Autodesk Fusion 360 part; units mm, degrees
(part 2 of 2)
sketch "Sketch14" plane through (0, 0, 0) normal (0, 0, 1) x (-1, 0, 0)
  spline S0 degree 5 poles (1.1125, -9.059) (1.0978, -9.0455) (1.0555, -9.011) (1.011, -8.9912) (0.9641, -8.9931) (0.9095, -9.0155) (0.8665, -9.0398) (0.8607, -9.0432) knots 0.525573 0.525573 0.525573 0.525573 0.525573 0.525573 0.528205 0.533333 0.534119 0.534119 0.534119 0.534119 0.534119 0.534119
  arc A0 (1.1125, -9.059) -> (0.8607, -9.0432) centre (0.8856, -10.654) ccw
  arc A1 (-0.4184, -9.7079) -> (2.3934, -10.0866) centre (0.8856, -10.654) ccw
  spline S1 degree 5 poles (0.6709, 13.445) (0.783, 13.4498) (1.0072, 13.459) (1.3442, 13.4715) (1.7958, 13.4859) (2.365, 13.4975) (2.9391, 13.4984) (3.5187, 13.4833) (4.106, 13.4469) (4.7062, 13.3844) (5.3283, 13.2926) (5.9822, 13.1694) (6.6768, 13.0129) (7.4173, 12.8216) (8.2027, 12.5932) (9.0235, 12.3247) (9.8597, 12.0116) (10.6769, 11.6473) (11.4304, 11.2245) (12.0725, 10.7371) (12.5591, 10.1826) (12.8561, 9.5641) (12.9463, 8.892) (12.8356, 8.1865) (12.5616, 7.4801) (12.1923, 6.8157) (11.8085, 6.235) (11.4898, 5.7696) (11.2987, 5.4297) (11.2671, 5.1966) (11.3773, 5.0079) (11.5611, 4.7626) (11.7362, 4.3632) (11.8325, 3.7477) (11.8251, 2.9297) (11.7255, 1.9782) (11.5691, 0.9945) (11.4045, 0.0892) (11.2826, -0.6397) (11.2442, -1.1314) (11.3109, -1.3806) (11.4696, -1.4712) (11.6758, -1.5583) (11.8871, -1.7597) (12.0894, -2.0706) (12.2879, -2.4194) (12.4965, -2.7197) (12.728, -2.9335) (12.9875, -3.0981) (13.2749, -3.2834) (13.5856, -3.566) (13.912, -3.9925) (14.2441, -4.5797) (14.5698, -5.3213) (14.8753, -6.1921) (15.1462, -7.1536) (15.3673, -8.1587) (15.5233, -9.1573) (15.5998, -10.1003) (15.5828, -10.9464) (15.4608, -11.6626) (15.2255, -12.2237) (14.8731, -12.6119) (14.4066, -12.8168) (13.8357, -12.8345) (13.1799, -12.6674) (12.4665, -12.3245) (11.7278, -11.8208) (10.9984, -11.1782) (10.3118, -10.4256) (9.698, -9.5988) (9.1805, -8.7406) (8.7731, -7.9018) (8.4778, -7.1402) (8.2807, -6.5221) (8.1557, -6.1073) (8.0671, -5.9319) (7.9735, -5.9948) (7.8294, -6.2361) (7.593, -6.5406) (7.2472, -6.7929) (6.8148, -6.9181) (6.383, -6.9377) (6.0614, -6.9338) (5.9338, -7.0029) (6.0018, -7.2066) (6.1645, -7.543) (6.2897, -7.972) (6.2688, -8.4304) (6.0758, -8.8508) (5.7419, -9.1752) (5.3303, -9.3696) (4.9133, -9.4359) (4.5448, -9.4322) (4.2529, -9.4431) (4.0374, -9.5402) (3.8635, -9.7382) (3.6665, -9.976) (3.3863, -10.167) (3.0517, -10.228) (2.7549, -10.1966) (2.5418, -10.1395) (2.4216, -10.0971) (2.3934, -10.0866) knots 0 0 0 0 0 0 0.00512821 0.01025641 0.01538462 0.02051282 0.02564103 0.03076923 0.03589744 0.04102564 0.04615385 0.05128205 0.05641026 0.06153846 0.06666667 0.07179487 0.07692308 0.08205128 0.08717949 0.09230769 0.0974359 0.1025641 0.10769231 0.11282051 0.11794872 0.12307692 0.12820513 0.13333333 0.13846154 0.14358974 0.14871795 0.15384615 0.15897436 0.16410256 0.16923077 0.17435897 0.17948718 0.18461538 0.18974359 0.19487179 0.2 0.20512821 0.21025641 0.21538462 0.22051282 0.22564103 0.23076923 0.23589744 0.24102564 0.24615385 0.25128205 0.25641026 0.26153846 0.26666667 0.27179487 0.27692308 0.28205128 0.28717949 0.29230769 0.2974359 0.3025641 0.30769231 0.31282051 0.31794872 0.32307692 0.32820513 0.33333333 0.33846154 0.34358974 0.34871795 0.35384615 0.35897436 0.36410256 0.36923077 0.37435897 0.37948718 0.38461538 0.38974359 0.39487179 0.4 0.40512821 0.41025641 0.41538462 0.42051282 0.42564103 0.43076923 0.43589744 0.44102564 0.44615385 0.45128205 0.45641026 0.46153846 0.46666667 0.47179487 0.47692308 0.48205128 0.48717949 0.49230769 0.4974359 0.5025641 0.50413901 0.50413901 0.50413901 0.50413901 0.50413901 0.50413901
  spline S2 degree 5 poles (-0.4184, -9.7079) (-0.4947, -9.7289) (-0.7038, -9.7805) (-1.0694, -9.8432) (-1.6197, -9.8735) (-2.3378, -9.8023) (-3.0366, -9.6007) (-3.5622, -9.2992) (-3.8526, -8.9306) (-3.8934, -8.5294) (-3.7467, -8.1242) (-3.5327, -7.7352) (-3.3803, -7.3754) (-3.3923, -7.0507) (-3.5931, -6.7603) (-3.9282, -6.4983) (-4.3136, -6.2565) (-4.6678, -6.0275) (-4.9601, -5.8076) (-5.2168, -5.597) (-5.4892, -5.3975) (-5.8342, -5.2103) (-6.2852, -5.0334) (-6.85, -4.8615) (-7.5179, -4.6873) (-8.2646, -4.5017) (-9.0581, -4.2949) (-9.8636, -4.057) (-10.6488, -3.7787) (-11.3903, -3.4522) (-12.0729, -3.0716) (-12.6879, -2.6335) (-13.2319, -2.1373) (-13.7056, -1.5858) (-14.1121, -0.9858) (-14.4558, -0.3482) (-14.7408, 0.3111) (-14.9701, 0.9713) (-15.1451, 1.61) (-15.2662, 2.2059) (-15.332, 2.7413) (-15.3397, 3.2051) (-15.2847, 3.5952) (-15.1607, 3.9217) (-14.9606, 4.1992) (-14.6768, 4.4397) (-14.3026, 4.644) (-13.8328, 4.7975) (-13.2671, 4.8789) (-12.6118, 4.8662) (-11.8835, 4.7446) (-11.1103, 4.5126) (-10.3365, 4.1907) (-9.6195, 3.8228) (-9.017, 3.4646) (-8.5761, 3.1758) (-8.321, 3.0107) (-8.2437, 3.0092) (-8.2866, 3.1872) (-8.3535, 3.5308) (-8.3608, 4.0006) (-8.2888, 4.5302) (-8.1739, 5.0419) (-8.076, 5.4679) (-8.0543, 5.7687) (-8.1385, 5.9551) (-8.3064, 6.1019) (-8.5111, 6.3) (-8.7096, 6.603) (-8.8732, 7.0146) (-8.9811, 7.5114) (-9.0199, 8.0542) (-8.9803, 8.6054) (-8.8551, 9.142) (-8.6396, 9.6517) (-8.3323, 10.1301) (-7.9349, 10.5777) (-7.4531, 10.9973) (-6.897, 11.39) (-6.2807, 11.7543) (-5.6208, 12.0873) (-4.9348, 12.3852) (-4.24, 12.6443) (-3.5517, 12.8619) (-2.8818, 13.0371) (-2.2375, 13.1714) (-1.6203, 13.2697) (-1.0271, 13.3388) (-0.4523, 13.3865) (-0.0014, 13.4134) (0.3348, 13.4302) (0.5588, 13.4402) (0.6709, 13.445) knots 0.55074943 0.55074943 0.55074943 0.55074943 0.55074943 0.55074943 0.55384615 0.55897436 0.56410256 0.56923077 0.57435897 0.57948718 0.58461538 0.58974359 0.59487179 0.6 0.60512821 0.61025641 0.61538462 0.62051282 0.62564103 0.63076923 0.63589744 0.64102564 0.64615385 0.65128205 0.65641026 0.66153846 0.66666667 0.67179487 0.67692308 0.68205128 0.68717949 0.69230769 0.6974359 0.7025641 0.70769231 0.71282051 0.71794872 0.72307692 0.72820513 0.73333333 0.73846154 0.74358974 0.74871795 0.75384615 0.75897436 0.76410256 0.76923077 0.77435897 0.77948718 0.78461538 0.78974359 0.79487179 0.8 0.80512821 0.81025641 0.81538462 0.82051282 0.82564103 0.83076923 0.83589744 0.84102564 0.84615385 0.85128205 0.85641026 0.86153846 0.86666667 0.87179487 0.87692308 0.88205128 0.88717949 0.89230769 0.8974359 0.9025641 0.90769231 0.91282051 0.91794872 0.92307692 0.92820513 0.93333333 0.93846154 0.94358974 0.94871795 0.95384615 0.95897436 0.96410256 0.96923077 0.97435897 0.97948718 0.98461538 0.98974359 0.99487179 1 1 1 1 1 1
  spline S3 degree 5 poles (10.4394, 5.8235) (10.3931, 5.7881) (10.3072, 5.7354) (10.2004, 5.7112) (10.1035, 5.785) (10.0524, 6.0062) (10.0679, 6.2608) (10.1457, 6.4583) (10.276, 6.5881) (10.4422, 6.7232) (10.6238, 6.9388) (10.798, 7.2554) (10.9418, 7.6564) (11.033, 8.1055) (11.0519, 8.5657) (10.9829, 9.0135) (10.8159, 9.4338) (10.5477, 9.8191) (10.183, 10.1666) (9.737, 10.4763) (9.232, 10.7498) (8.6932, 10.9903) (8.1445, 11.2016) (7.6044, 11.3882) (7.0817, 11.5544) (6.5725, 11.7038) (6.064, 11.8395) (5.5378, 11.9626) (4.9738, 12.0728) (4.3532, 12.1672) (3.6623, 12.2402) (2.8937, 12.2836) (2.046, 12.2882) (1.1234, 12.2444) (0.1362, 12.1433) (-0.8999, 11.9781) (-1.9636, 11.7445) (-3.028, 11.4421) (-4.0609, 11.0754) (-5.0246, 10.655) (-5.8791, 10.1958) (-6.5871, 9.7149) (-7.1181, 9.2293) (-7.4527, 8.7537) (-7.5871, 8.2979) (-7.5371, 7.8656) (-7.3442, 7.4499) (-7.0721, 7.0381) (-6.7926, 6.6227) (-6.575, 6.2119) (-6.4734, 5.8389) (-6.5142, 5.5763) (-6.6952, 5.5032) (-6.9871, 5.6548) (-7.3363, 5.9913) (-7.6804, 6.4335) (-7.9627, 6.8924) (-8.1447, 7.2973) (-8.2249, 7.6326) (-8.2277, 7.927) (-8.1839, 8.225) (-8.1112, 8.5625) (-7.9999, 8.9459) (-7.8259, 9.3632) (-7.5619, 9.7916) (-7.1885, 10.2065) (-6.7064, 10.5903) (-6.1327, 10.9327) (-5.495, 11.2287) (-4.8255, 11.4786) (-4.1554, 11.6858) (-3.5096, 11.8567) (-2.9001, 11.9989) (-2.324, 12.1204) (-1.769, 12.2289) (-1.2172, 12.3309) (-0.6494, 12.4306) (-0.0486, 12.5293) (0.5947, 12.6243) (1.2817, 12.7088) (2.0075, 12.7742) (2.7633, 12.8105) (3.5375, 12.8087) (4.3183, 12.7612) (5.0947, 12.6639) (5.8593, 12.5171) (6.6085, 12.3265) (7.3404, 12.1002) (8.0535, 11.8474) (8.7448, 11.5763) (9.4085, 11.292) (10.0336, 10.9948) (10.603, 10.6783) (11.0915, 10.3274) (11.4718, 9.9244) (11.7195, 9.4547) (11.8193, 8.9124) (11.7697, 8.3061) (11.5905, 7.6658) (11.3195, 7.0395) (11.0033, 6.4823) (10.7528, 6.1345) (10.585, 5.9477) (10.4857, 5.8589) (10.4394, 5.8235) knots 0 0 0 0 0 0 0.01 0.02 0.03 0.04 0.05 0.06 0.07 0.08 0.09 0.1 0.11 0.12 0.13 0.14 0.15 0.16 0.17 0.18 0.19 0.2 0.21 0.22 0.23 0.24 0.25 0.26 0.27 0.28 0.29 0.3 0.31 0.32 0.33 0.34 0.35 0.36 0.37 0.38 0.39 0.4 0.41 0.42 0.43 0.44 0.45 0.46 0.47 0.48 0.49 0.5 0.51 0.52 0.53 0.54 0.55 0.56 0.57 0.58 0.59 0.6 0.61 0.62 0.63 0.64 0.65 0.66 0.67 0.68 0.69 0.7 0.71 0.72 0.73 0.74 0.75 0.76 0.77 0.78 0.79 0.8 0.81 0.82 0.83 0.84 0.85 0.86 0.87 0.88 0.89 0.9 0.91 0.92 0.93 0.94 0.95 0.96 0.97 0.98 0.99 1 1 1 1 1 1
  spline S4 degree 5 poles (-2.7641, 6.897) (-2.7136, 6.906) (-2.6132, 6.9126) (-2.4675, 6.8873) (-2.2919, 6.7846) (-2.1215, 6.5566) (-2.0143, 6.253) (-1.979, 5.9039) (-2.0187, 5.5426) (-2.13, 5.2031) (-2.3042, 4.9174) (-2.5274, 4.7132) (-2.7812, 4.611) (-3.0426, 4.6214) (-3.2849, 4.7423) (-3.4812, 4.9614) (-3.6078, 5.258) (-3.6483, 5.6047) (-3.5975, 5.9692) (-3.4636, 6.316) (-3.2638, 6.6104) (-3.0698, 6.7793) (-2.9167, 6.8582) (-2.8147, 6.8879) (-2.7641, 6.897) knots 0 0 0 0 0 0 0.05 0.1 0.15 0.2 0.25 0.3 0.35 0.4 0.45 0.5 0.55 0.6 0.65 0.7 0.75 0.8 0.85 0.9 0.95 1 1 1 1 1 1
  spline S5 degree 5 poles (0.1879, -7.9704) (0.1651, -8.0236) (0.1127, -8.1288) (0.0145, -8.2815) (-0.1505, -8.4695) (-0.3928, -8.6711) (-0.649, -8.8363) (-0.8999, -8.9645) (-1.1327, -9.056) (-1.3474, -9.109) (-1.5548, -9.1205) (-1.7679, -9.0879) (-1.9955, -9.0109) (-2.2349, -8.893) (-2.4648, -8.7438) (-2.654, -8.5757) (-2.7693, -8.4013) (-2.784, -8.2307) (-2.6874, -8.0683) (-2.4886, -7.9117) (-2.209, -7.7561) (-1.8773, -7.5965) (-1.524, -7.4315) (-1.1753, -7.2662) (-0.848, -7.1154) (-0.5519, -6.9989) (-0.2926, -6.9377) (-0.0733, -6.9485) (0.102, -7.0404) (0.2264, -7.2089) (0.2901, -7.4367) (0.2857, -7.6474) (0.2492, -7.8099) (0.2106, -7.9173) (0.1879, -7.9704) knots 0 0 0 0 0 0 0.033333 0.066667 0.1 0.133333 0.166667 0.2 0.233333 0.266667 0.3 0.333333 0.366667 0.4 0.433333 0.466667 0.5 0.533333 0.566667 0.6 0.633333 0.666667 0.7 0.733333 0.766667 0.8 0.833333 0.866667 0.9 0.933333 0.966667 1 1 1 1 1 1
  line L0 (5, 6) -> (5.5551, 6.9506)
  spline S6 degree 5 poles (5.5551, 6.9506) (5.5848, 6.9597) (5.6705, 6.983) (5.8179, 7.0105) (6.0309, 7.0215) (6.297, 6.972) (6.5506, 6.8162) (6.7385, 6.5461) (6.8412, 6.1684) (6.8505, 5.7228) (6.7682, 5.2711) (6.6041, 4.8826) (6.3745, 4.621) (6.1008, 4.5319) (5.8082, 4.6262) (5.5241, 4.8758) (5.2754, 5.2304) (5.1244, 5.5494) (5.0469, 5.7823) (5.0127, 5.9292) (5, 6) knots 0.222701 0.222701 0.222701 0.222701 0.222701 0.222701 0.25 0.3 0.35 0.4 0.45 0.5 0.55 0.6 0.65 0.7 0.75 0.8 0.85 0.9 0.95 1 1 1 1 1 1
  spline S7 degree 5 poles (3.5692, -6.8433) (3.6043, -6.856) (3.6794, -6.8823) (3.8061, -6.9223) (4.0002, -6.9732) (4.272, -7.0356) (4.5557, -7.1066) (4.8314, -7.1988) (5.078, -7.3226) (5.2745, -7.4814) (5.4018, -7.6695) (5.4448, -7.8747) (5.3954, -8.08) (5.2543, -8.2649) (5.0345, -8.4072) (4.7587, -8.4857) (4.4547, -8.4836) (4.1514, -8.3912) (3.8746, -8.2093) (3.6428, -7.9535) (3.4638, -7.6549) (3.3387, -7.3522) (3.2642, -7.085) (3.2356, -6.8859) (3.2489, -6.7742) (3.3043, -6.7465) (3.3855, -6.7726) (3.4687, -6.8057) (3.5341, -6.8305) (3.5692, -6.8433) knots 0 0 0 0 0 0 0.04 0.08 0.12 0.16 0.2 0.24 0.28 0.32 0.36 0.4 0.44 0.48 0.52 0.56 0.6 0.64 0.68 0.72 0.76 0.8 0.84 0.88 0.92 0.96 1 1 1 1 1 1
  spline S8 degree 5 poles (-1, -6) (-0.9263, -6.0109) (-0.7895, -6.0343) (-0.6205, -6.0771) (-0.4842, -6.1578) (-0.4887, -6.306) (-0.668, -6.4812) (-0.9946, -6.6344) (-1.4281, -6.7112) (-1.9261, -6.6683) (-2.4575, -6.4946) (-3.0012, -6.2043) (-3.5444, -5.829) (-4.0813, -5.41) (-4.6112, -4.9909) (-5.1372, -4.6101) (-5.6643, -4.2919) (-6.1984, -4.0456) (-6.7457, -3.8685) (-7.3116, -3.7479) (-7.9003, -3.6638) (-8.5133, -3.5904) (-9.1491, -3.4994) (-9.8027, -3.3614) (-10.4661, -3.1491) (-11.1286, -2.8397) (-11.7772, -2.4174) (-12.3971, -1.8764) (-12.9722, -1.2226) (-13.485, -0.4774) (-13.9176, 0.321) (-14.2533, 1.1246) (-14.4786, 1.8814) (-14.5849, 2.5424) (-14.5707, 3.0681) (-14.4432, 3.4348) (-14.2199, 3.6411) (-13.9316, 3.7154) (-13.6114, 3.7012) (-13.2853, 3.6437) (-12.9596, 3.573) (-12.6234, 3.5017) (-12.2587, 3.4296) (-11.8475, 3.346) (-11.3819, 3.2332) (-10.8645, 3.0705) (-10.3054, 2.8387) (-9.7219, 2.525) (-9.136, 2.1272) (-8.5732, 1.6582) (-8.061, 1.1516) (-7.626, 0.6569) (-7.2904, 0.231) (-7.0689, -0.0691) (-6.9653, -0.194) (-6.9691, -0.1095) (-7.0534, 0.1966) (-7.1826, 0.7135) (-7.318, 1.4065) (-7.4251, 2.2144) (-7.4779, 3.0523) (-7.4606, 3.8283) (-7.368, 4.4571) (-7.2077, 4.8751) (-7.0005, 5.0541) (-6.783, 5.0174) (-6.6072, 4.851) (-6.5178, 4.6493) (-6.5225, 4.4413) (-6.5897, 4.1849) (-6.6736, 3.8184) (-6.7343, 3.3035) (-6.747, 2.642) (-6.6972, 1.8607) (-6.5805, 1.0045) (-6.4002, 0.1272) (-6.1658, -0.717) (-5.891, -1.4828) (-5.5925, -2.1418) (-5.2881, -2.6922) (-4.9938, -3.1506) (-4.7223, -3.5442) (-4.4794, -3.9025) (-4.2626, -4.2496) (-4.0577, -4.5955) (-3.8386, -4.9308) (-3.5766, -5.2374) (-3.2488, -5.4951) (-2.8457, -5.6895) (-2.3805, -5.8212) (-1.8841, -5.9021) (-1.4961, -5.9422) (-1.2317, -5.9692) (-1.0737, -5.9891) (-1, -6) knots 0 0 0 0 0 0 0.01111111 0.02222222 0.03333333 0.04444444 0.05555556 0.06666667 0.07777778 0.08888889 0.1 0.11111111 0.12222222 0.13333333 0.14444444 0.15555556 0.16666667 0.17777778 0.18888889 0.2 0.21111111 0.22222222 0.23333333 0.24444444 0.25555556 0.26666667 0.27777778 0.28888889 0.3 0.31111111 0.32222222 0.33333333 0.34444444 0.35555556 0.36666667 0.37777778 0.38888889 0.4 0.41111111 0.42222222 0.43333333 0.44444444 0.45555556 0.46666667 0.47777778 0.48888889 0.5 0.51111111 0.52222222 0.53333333 0.54444444 0.55555556 0.56666667 0.57777778 0.58888889 0.6 0.61111111 0.62222222 0.63333333 0.64444444 0.65555556 0.66666667 0.67777778 0.68888889 0.7 0.71111111 0.72222222 0.73333333 0.74444444 0.75555556 0.76666667 0.77777778 0.78888889 0.8 0.81111111 0.82222222 0.83333333 0.84444444 0.85555556 0.86666667 0.87777778 0.88888889 0.9 0.91111111 0.92222222 0.93333333 0.94444444 0.95555556 0.96666667 0.97777778 0.98888889 1 1 1 1 1 1
  spline S9 degree 5 poles (10, -2) (10.01, -2.036) (10.0453, -2.1108) (10.1474, -2.2349) (10.3859, -2.4339) (10.8347, -2.7499) (11.393, -3.1342) (12.0076, -3.5812) (12.6229, -4.0819) (13.1891, -4.627) (13.6733, -5.2111) (14.0597, -5.8323) (14.3455, -6.4896) (14.5375, -7.1809) (14.6486, -7.9014) (14.6949, -8.6414) (14.692, -9.3839) (14.6517, -10.1032) (14.5784, -10.7623) (14.471, -11.3191) (14.3252, -11.735) (14.1362, -11.9825) (13.9007, -12.0521) (13.6202, -11.9628) (13.3012, -11.7594) (12.9526, -11.4943) (12.5846, -11.2134) (12.206, -10.9382) (11.8235, -10.6576) (11.4425, -10.342) (11.068, -9.9532) (10.7055, -9.4558) (10.3621, -8.8276) (10.047, -8.0724) (9.7717, -7.2242) (9.5468, -6.3366) (9.3788, -5.4754) (9.2683, -4.7097) (9.2065, -4.1044) (9.1724, -3.7107) (9.1314, -3.5595) (9.029, -3.6505) (8.804, -3.9529) (8.4136, -4.4136) (7.8609, -4.9623) (7.1905, -5.5211) (6.4714, -6.0135) (5.7845, -6.3744) (5.2082, -6.559) (4.8035, -6.5535) (4.6023, -6.3818) (4.5875, -6.1225) (4.7071, -5.8806) (4.9057, -5.7334) (5.1562, -5.676) (5.452, -5.6487) (5.794, -5.5768) (6.1761, -5.4127) (6.5828, -5.1473) (6.9941, -4.7946) (7.3893, -4.384) (7.7508, -3.9497) (8.0681, -3.5212) (8.3413, -3.1136) (8.5775, -2.7318) (8.7882, -2.3723) (8.9859, -2.0258) (9.1813, -1.6798) (9.3801, -1.3213) (9.5834, -0.938) (9.7877, -0.5199) (9.9851, -0.061) (10.1642, 0.4399) (10.3094, 0.9769) (10.405, 1.5388) (10.4387, 2.1108) (10.405, 2.676) (10.3098, 3.2174) (10.1726, 3.7193) (10.0326, 4.169) (9.9371, 4.5561) (9.9267, 4.87) (10.0234, 5.0985) (10.2124, 5.225) (10.4434, 5.2306) (10.6607, 5.1043) (10.8309, 4.853) (10.9445, 4.4982) (11.0055, 4.0669) (11.0259, 3.5855) (11.0179, 3.0709) (10.9923, 2.533) (10.9576, 1.978) (10.9188, 1.4115) (10.8765, 0.8411) (10.8256, 0.2797) (10.7543, -0.2508) (10.6494, -0.7257) (10.5042, -1.1234) (10.3248, -1.4329) (10.1363, -1.6588) (10.0217, -1.7964) (9.9855, -1.8949) (9.99, -1.964) (10, -2) knots 0 0 0 0 0 0 0.01 0.02 0.03 0.04 0.05 0.06 0.07 0.08 0.09 0.1 0.11 0.12 0.13 0.14 0.15 0.16 0.17 0.18 0.19 0.2 0.21 0.22 0.23 0.24 0.25 0.26 0.27 0.28 0.29 0.3 0.31 0.32 0.33 0.34 0.35 0.36 0.37 0.38 0.39 0.4 0.41 0.42 0.43 0.44 0.45 0.46 0.47 0.48 0.49 0.5 0.51 0.52 0.53 0.54 0.55 0.56 0.57 0.58 0.59 0.6 0.61 0.62 0.63 0.64 0.65 0.66 0.67 0.68 0.69 0.7 0.71 0.72 0.73 0.74 0.75 0.76 0.77 0.78 0.79 0.8 0.81 0.82 0.83 0.84 0.85 0.86 0.87 0.88 0.89 0.9 0.91 0.92 0.93 0.94 0.95 0.96 0.97 0.98 0.99 1 1 1 1 1 1
  spline S10 degree 5 poles (2.6568, -7.8631) (2.6953, -7.8921) (2.772, -7.9484) (2.8852, -8.0273) (3.0274, -8.1223) (3.1793, -8.2345) (3.2947, -8.3544) (3.3652, -8.4941) (3.3848, -8.6583) (3.3514, -8.8381) (3.2663, -9.0161) (3.1342, -9.1712) (2.9634, -9.2832) (2.7654, -9.3383) (2.5547, -9.3331) (2.347, -9.2713) (2.1572, -9.1614) (1.997, -9.0139) (1.8734, -8.8386) (1.7867, -8.6421) (1.7319, -8.4293) (1.7018, -8.2049) (1.6893, -7.9757) (1.689, -7.7516) (1.7005, -7.5485) (1.728, -7.3863) (1.778, -7.284) (1.8566, -7.2545) (1.9673, -7.2994) (2.1089, -7.4057) (2.2766, -7.5516) (2.4255, -7.6805) (2.541, -7.7744) (2.6183, -7.8341) (2.6568, -7.8631) knots 0 0 0 0 0 0 0.033333 0.066667 0.1 0.133333 0.166667 0.2 0.233333 0.266667 0.3 0.333333 0.366667 0.4 0.433333 0.466667 0.5 0.533333 0.566667 0.6 0.633333 0.666667 0.7 0.733333 0.766667 0.8 0.833333 0.866667 0.9 0.933333 0.966667 1 1 1 1 1 1
  spline S11 degree 5 poles (2, 8) (2.0408, 7.9847) (2.1215, 7.9515) (2.2388, 7.8934) (2.3822, 7.7987) (2.5224, 7.6479) (2.6058, 7.4628) (2.6178, 7.2467) (2.5509, 7.0115) (2.407, 6.7785) (2.195, 6.5726) (1.9298, 6.4191) (1.6308, 6.3382) (1.3211, 6.3412) (1.0257, 6.4261) (0.7697, 6.5807) (0.5747, 6.7864) (0.4571, 7.0213) (0.4247, 7.2632) (0.474, 7.4933) (0.591, 7.6973) (0.7571, 7.8649) (0.9523, 7.9897) (1.1599, 8.0696) (1.3709, 8.1063) (1.5823, 8.1045) (1.751, 8.0767) (1.8766, 8.0431) (1.9592, 8.0153) (2, 8) knots 0 0 0 0 0 0 0.04 0.08 0.12 0.16 0.2 0.24 0.28 0.32 0.36 0.4 0.44 0.48 0.52 0.56 0.6 0.64 0.68 0.72 0.76 0.8 0.84 0.88 0.92 0.96 1 1 1 1 1 1
  circle A2 centre (0.8856, -10.654) radius 0.9124
  constraint concentric A0 A2
hole "Hole1" at (-0.8856, 10.654, 0) direction (0, 0, -1) diameter 2 depth 3 tip angle 118 bodies 1
